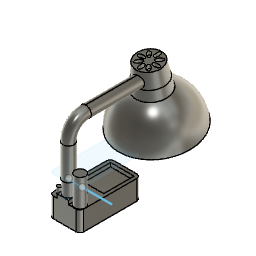
Project D1 (Autodesk Fusion 360 design; units mm, degrees)
Autodesk Fusion 360 part; units mm, degrees
sketch "Sketch1" plane through (0, 0, 0) normal (0, 1, 0) x (1, 0, 0)
sketch "Sketch2" plane through (0, 0, 0) normal (0, 0, 1) x (1, 0, 0)
  line L0 (0, 160) -> (80, 160)
  line L1 (80, 160) -> (80, 0)
  line L2 (80, 0) -> (0, 0)
  line L3 (0, 0) -> (0, 160)
  dimension "d1" = 80
  dimension "d2" = 160
  constraint horizontal L0
  constraint vertical L1
  constraint horizontal L2
  constraint vertical L3
  measures "d1" distance of L0.start L0.end
  measures "d2" distance of L0.start L2.end
extrude "Extrude1" add sketch "Sketch2" against normal blind 27 makes body 1
fillet "Fillet1" radius 10 3 edges at (80, 160, -13.5) (80, 0, -13.5) (0, 160, -13.5) on bodies 1
fillet "Fillet2" radius 10 1 edges at (0, 0, -13.5) on bodies 1
sketch "Sketch3" plane through (0, 0, 0) normal (0, 0, 1) x (-1, 0, 0)
  arc A0 (0, -10) -> (-10, 0) centre (-10, -10) ccw
  line L0 (-10, 0) -> (-70, 0)
  arc A1 (-70, 0) -> (-80, -10) centre (-70, -10) ccw
  line L1 (-80, -10) -> (-80, -150)
  arc A2 (-80, -150) -> (-70, -160) centre (-70, -150) ccw
  line L2 (-70, -160) -> (-10, -160)
  arc A3 (-10, -160) -> (0, -150) centre (-10, -150) ccw
  line L3 (0, -150) -> (0, -10)
sketch "Sketch4" plane through (0, 0, 0) normal (0, 0, 1) x (-1, 0, 0)
  line L0 (-71.3132, -71.4345) -> (-9.3132, -71.4345)
  line L1 (-9.3132, -71.4345) -> (-9.3132, -151.4345)
  line L2 (-9.3132, -151.4345) -> (-71.3132, -151.4345)
  line L3 (-71.3132, -151.4345) -> (-71.3132, -71.4345)
  dimension "d9" = 62
  dimension "d10" = 80
  constraint horizontal L0
  constraint vertical L1
  constraint horizontal L2
  constraint vertical L3
  measures "d9" distance of L0.start L0.end
  measures "d10" distance of L0.start L2.end
extrude "Extrude2" cut sketch "Sketch4" against normal blind 10 bodies 1
sketch "Sketch5" plane through (0, 0, 0) normal (0, 0, 1) x (1, 0, 0)
  circle A0 centre (65.5404, 14.9529) radius 14
  dimension "d13" = 28
  measures "d13" diameter of A0
extrude "Extrude3" add sketch "Sketch5" along normal blind 40 bodies 1
sketch "Sketch6" plane through (0, 0, 0) normal (0, 0, 1) x (1, 0, 0)
  line L0 (50, 0) -> (20, 0)
  line L1 (20, 0) -> (20, 50)
  line L2 (20, 50) -> (50, 50)
  line L3 (50, 50) -> (50, 0)
  dimension "d16" = 30
  constraint horizontal L0
  constraint vertical L1
  constraint horizontal L2
  constraint vertical L3
  measures "d16" distance of L0.start L0.end
extrude "Extrude4" add sketch "Sketch6" along normal blind 10 bodies 1
sketch "Sketch7" plane through (0, 0, 10) normal (0, 0, 1) x (-1, 0, 0)
  line L0 (-50, -50) -> (-20, -50)
  line L1 (-20, -50) -> (-20, 0)
  line L2 (-20, 0) -> (-50, 0)
  line L3 (-50, 0) -> (-50, -50)
  circle A0 centre (-35.247, -15.3012) radius 14
  dimension "d19" = 28
  measures "d19" diameter of A0
extrude "Extrude5" add sketch "Sketch7" along normal blind 15 contours A0 bodies 1
sketch "Sketch8" plane through (0, 0, 0) normal (0, 0, 1) x (1, 0, 0)
  circle A0 centre (10, 15) radius 5
  dimension "d22" = 10
  measures "d22" diameter of A0
extrude "Extrude6" add sketch "Sketch8" along normal blind 15 bodies 1
sketch "Sketch9" plane through (0, 0, 0) normal (0, 0, 1) x (1, 0, 0)
  line L0 (9.8673, 32.5058) -> (9.8673, 32.5058)
  line L1 (7.8673, 34.5058) -> (7.8673, 44.5058)
  line L2 (9.8673, 46.5058) -> (9.8673, 46.5058)
  line L3 (11.8673, 44.5058) -> (11.8673, 34.5058)
  arc A0 (9.8673, 32.5058) -> (11.8673, 34.5058) centre (9.8673, 34.5058) ccw
  arc A1 (7.8673, 34.5058) -> (9.8673, 32.5058) centre (9.8673, 34.5058) ccw
  arc A2 (11.8673, 44.5058) -> (9.8673, 46.5058) centre (9.8673, 44.5058) ccw
  arc A3 (9.8673, 46.5058) -> (7.8673, 44.5058) centre (9.8673, 44.5058) ccw
  point P0 (11.8673, 32.5058)
  point P1 (7.8673, 32.5058)
  point P2 (11.8673, 46.5058)
  dimension "d25" = 4
  dimension "d26" = 14
  dimension "d27" = 2
  dimension "d28" = 2
  dimension "d29" = 2
  constraint vertical L1
  constraint vertical L3
  constraint coincident P0 L3
  constraint tangent L3 A0
  constraint coincident P1 L0
  constraint coincident P1 L1
  constraint tangent L1 A1
  constraint coincident P2 L3
  constraint tangent L3 A2
  constraint tangent L1 A3
  constraint equal A2 A3
  measures "d25" distance of P0 P1
  measures "d26" distance of P0 P2
  measures "d27" radius of A0
  measures "d28" radius of A1
  measures "d29" radius of A2
extrude "Extrude7" cut sketch "Sketch9" against normal blind 7 bodies 1
sketch "Sketch10" plane through (0, 0, 10) normal (0, 0, 1) x (-1, 0, 0)
  circle A0 centre (-35.247, -15.3012) radius 14
  line L0 (-50, -50) -> (-20, -50)
  line L1 (-20, -50) -> (-20, 0)
  line L2 (-20, 0) -> (-50, 0)
  line L3 (-50, 0) -> (-50, -50)
  line L4 (-31, -45) -> (-39, -45)
  line L5 (-39, -45) -> (-39, -35)
  line L6 (-39, -35) -> (-31, -35)
  line L7 (-31, -35) -> (-31, -45)
  dimension "d32" = 8
  dimension "d33" = 10
  constraint horizontal L4
  constraint vertical L5
  constraint horizontal L6
  constraint vertical L7
  measures "d32" distance of L4.start L4.end
  measures "d33" distance of L4.start L6.end
extrude "Extrude8" cut sketch "Sketch10" against normal blind 7 contours L4 L5 L6 L7 bodies 1
sketch "Sketch11" plane through (0, 0, 0) normal (1, 0, 0) x (0, 1, 0)
  line L0 (16.2634, 104.9165) -> (1.2634, 104.9165)
  line L1 (1.2634, 104.9165) -> (1.2634, 39.9165)
  line L2 (1.2634, 39.9165) -> (16.2634, 39.9165)
  line L3 (16.2634, 39.9165) -> (16.2634, 104.9165)
  line L4 (16.2634, 110.373) -> (16.2634, 35)
  dimension "d36" = 15
  dimension "d37" = 65
  constraint horizontal L0
  constraint vertical L1
  constraint horizontal L2
  constraint vertical L3
  constraint perpendicular L2 L4
  measures "d36" distance of L0.start L0.end
  measures "d37" distance of L0.start L2.end
revolve "Revolve1" add sketch "Sketch11" angle 360 about axis through (0, 16.2634, 110.373) along (0, 0, -1) separate body makes body 2
move_face "MoveFace1" to x (1, 0, 0) y (0, 1, 0) z (0, 0, 1) at (40, 0, 10) 1 faces at (0.7477, 1.282, 83.2498) on bodies 2
move_body "Move1" bodies 2 to x (1, 0, 0) y (0, 1, 0) z (0, 0, 1) at (-5, 0, -20)
sketch "Sketch12" plane through (0, 0, 0) normal (1, 0, 0) x (0, 1, 0)
sketch "Sketch13" plane through (0, 0, 0) normal (1, 0, 0) x (0, 1, 0)
sketch "Sketch14" plane through (0, 0, 0) normal (1, 0, 0) x (0, 1, 0)
  arc A0 (60, 122.9657) -> (17.0403, 79.284) centre (60, 80) ccw
pipe "Pipe1" add diameter 30 path "Sketch14" along A0 separate body makes body 3
move_face "MoveFace2" to x (1, 0, 0) y (0, 1, 0) z (0, 0, 1) at (0, -1, 0) 1 faces at (35.7477, 1.282, 63.2498) on bodies 2
move_face "MoveFace3" to x (1, 0, 0) y (0, 1, 0) z (0, 0, 1) at (0, -2, 2) 1 faces at (4.0626, 6.6698, 101.2421) on bodies 3
move_face "MoveFace4" to x (1, 0, 0) y (0, 1, 0) z (0, 0, 1) at (35, 0, 0) 1 faces at (-1.7653, 54.7653, 139.771) on bodies 3
extrude "Extrude9" add 1 faces at (30.0178, 60, 124.8543) along direction (0, 1, 0) blind 90 on bodies 3 bodies 3
extrude "Extrude10" add 1 faces at (26.6667, 56.6667, -27) along direction (0, 0, -1) blind 25 on bodies 1 bodies 1
sketch "Sketch15" plane through (0, 0, 0) normal (1, 0, 0) x (0, 1, 0)
sketch "Sketch16" plane through (0, 0, 0) normal (1, 0, 0) x (0, 1, 0)
  line L0 (282.5766, 151.0827) -> (279.0659, 177.8527)
  line L1 (282.5766, 151.0827) -> (308.0478, 151.0827) construction
  line L2 (279.0659, 177.8527) -> (273.8459, 217.5027)
  line L3 (279.0659, 177.8527) -> (317.4124, 177.8527) construction
  arc A0 (340, 60) -> (240, 160) centre (240, 60) ccw
  line L4 (240, 160) -> (240, 60)
  line L5 (240, 60) -> (340, 60)
  line L6 (282.5766, 151.0827) -> (240, 151.0827)
  line L7 (240, 180) -> (278.7832, 180)
  line L8 (273.8459, 217.5027) -> (240, 217.5027)
  line L9 (240, 217.5027) -> (240, 180)
  line L10 (240, 180) -> (240, 151.0827)
  line L11 (240, 240) -> (240, 50)
  dimension "d72" = 26.77
  constraint horizontal L1
  constraint horizontal L3
  constraint coincident A0.centre L4.end
  constraint perpendicular L4 L5
  constraint coincident L4 L6.end
  constraint perpendicular L4 L6
  constraint coincident L2 L7.end
  constraint parallel L6 L7
  constraint perpendicular L4 L8
  constraint perpendicular L7 L9
  constraint perpendicular L6 L10
  constraint perpendicular L5 L11
  measures "d72" vertical distance of L0.start L0.end
revolve "Revolve2" add sketch "Sketch16" angle 360 about axis through (0, 240, 240) along (0, 0, -1) separate body makes body 4
move_body "Move2" bodies 4 to x (1, 0, 0) y (0, 0.976296, 0.21644) z (0, -0.21644, 0.976296) at (0, 47.0867, -113.4516)
move_body "Move3" bodies 4 to x (1, 0, 0) y (0, 0.996195, -0.087156) z (0, 0.087156, 0.996195) at (0, 2.7825, 14.5845)
move_body "Move4" bodies 4 to x (1, 0, 0) y (0, 1, 0) z (0, 0, 1) at (0, -70, 10)
move_body "Move5" bodies 4 to x (1, 0, 0) y (0, 1, 0) z (0, 0, 1) at (32, 0, 0)
move_body "Move6" bodies 1 to x (1, 0, 0) y (0, 1, 0) z (0, 0, 1) at (0, 0, -50)
move_body "Move7" bodies 2 to x (1, 0, 0) y (0, 1, 0) z (0, 0, 1) at (0, 0, -25)
extrude "Extrude11" add 1 faces at (38.3611, 9.7448, 59.9165) along direction (0, 0, 1) blind 20 on bodies 2 bodies 2 4 3
move_body "Move8" bodies 4 to x (1, 0, 0) y (0, 1, 0) z (0, 0, 1) at (0, 50, 0)
extrude "Extrude12" add 1 faces at (67.8737, 10.9115, -10) along direction (0, 0, 1) blind 7 on bodies 1 bodies 1
extrude "Extrude13" add 1 faces at (30.0178, 150, 124.8543) along direction (0, 1, 0) blind 50 on bodies 2 bodies 2 4
sketch "Sketch17" plane through (0, -16.077, 122.1167) normal (0, -0.130526, 0.991445) x (1, 0, 0)
  circle A0 centre (32, 247.5539) radius 33.8459
  ellipse E0 centre (12.5438, 247.5239) end of major axis (22.1005, 247.5239) minor radius 5
  line L0 (2.987, 247.5239) -> (22.1005, 247.5239)
  line L1 (12.5438, 242.5239) -> (12.5438, 252.5239)
  dimension "d83" = 10
  constraint coincident E0 L0.start
  constraint coincident E0 L0.end
  constraint coincident E0 L1.start
  constraint coincident E0 L1.end
sketch "Sketch18" plane through (32, 229.359, 154.4289) normal (0, -0.130526, 0.991445) x (1, 0, 0)
extrude "Extrude14" add 1 faces at (39.8615, 9.6484, -25) along direction (0, 0, 1) blind 22 on bodies 1 bodies 1 2
extrude "Extrude15" add 1 faces at (67.8737, 10.9115, -3) along direction (0, 0, 1) blind 25 on bodies 1 bodies 1
sketch "Sketch19" plane through (0, 0, -40) normal (0, 0, 1) x (-1, 0, 0)
  line L0 (-39, -45) -> (-39, -35)
  line L1 (-39, -35) -> (-31, -35)
  line L2 (-31, -35) -> (-31, -45)
  line L3 (-31, -45) -> (-39, -45)
  circle A0 centre (-35.247, -15.3012) radius 14
  line L4 (-50, -50) -> (-20, -50)
  line L5 (-20, -50) -> (-20, 0)
  line L6 (-20, 0) -> (-50, 0)
  line L7 (-50, 0) -> (-50, -50)
  line L8 (0, -50) -> (0, -47.6437)
  line L9 (0, -47.6437) -> (-114.7068, -47.6437)
  line L10 (-114.7068, -47.6437) -> (-38.5734, -47.6437)
  constraint vertical L8
  constraint perpendicular L8 L9
  constraint parallel L9 L10
sketch "Sketch20" plane through (0, 0, 0) normal (0, 0, 1) x (1, 0, 0)
sketch "Sketch21" plane through (0, 0, 0) normal (1, 0, 0) x (0, 1, 0)
  line L0 (40, -30) -> (37.0787, -33.5355)
  arc A0 (40, -30) -> (45, -32.831) centre (45, -27) ccw
  line L1 (45, -32.831) -> (45, -36)
  line L2 (45, -36) -> (37, -36)
  line L3 (37, -36) -> (37.0787, -33.5355)
  constraint vertical L1
  constraint perpendicular L1 L2
extrude "Extrude16" add sketch "Sketch21" along normal blind 10 separate body makes body 5
move_body "Move9" bodies 5 to x (1, 0, 0) y (0, 1, 0) z (0, 0, 1) at (30, 0, -5.5)
sketch "Sketch22" plane through (32, 229.359, 154.4289) normal (0, -0.130526, 0.991445) x (1, 0, 0)
extrude "Extrude17" add sketch "Sketch17" along normal blind 1 contours E0 L0 L1 | E0 L0 L1 | E0 L0 L1 | E0 L0 L1 bodies 1
sketch "Sketch23" plane through (0, -16.077, 122.1167) normal (0, -0.130526, 0.991445) x (1, 0, 0)
  ellipse E0 centre (12.5438, 247.5239) end of major axis (22.1005, 247.5239) minor radius 5
  circle A0 centre (32, 247.5539) radius 33.8459
  ellipse E1 centre (52.1147, 247.0081) end of major axis (42.1147, 247.0081) minor radius 5
  line L0 (62.1147, 247.0081) -> (42.1147, 247.0081)
  line L1 (52.1147, 252.0081) -> (52.1147, 242.0081)
  ellipse E2 centre (18.9077, 260.8879) end of major axis (25.6653, 254.1303) minor radius 5
  ellipse E3 centre (32.3427, 270.0803) end of major axis (32.3427, 260.5236) minor radius 5
  ellipse E4 centre (46.1147, 262.0081) end of major axis (39.0436, 254.937) minor radius 5
  line L2 (53.1858, 269.0792) -> (39.0436, 254.937)
  line L3 (42.5792, 265.5436) -> (49.6502, 258.4726)
  ellipse E5 centre (32.3427, 227.0803) end of major axis (32.3427, 217.5236) minor radius 5
  ellipse E6 centre (18.1147, 234.0081) end of major axis (11.0436, 226.937) minor radius 5
  line L4 (25.1858, 241.0792) -> (11.0436, 226.937)
  line L5 (14.5792, 237.5436) -> (21.6502, 230.4726)
  ellipse E7 centre (45.9077, 232.8879) end of major axis (52.6653, 226.1303) minor radius 5
  dimension "d95" = 20
  dimension "d96" = 20
  dimension "d97" = 20
  constraint horizontal L0
  constraint coincident E1 L0.start
  constraint coincident E1 L0.end
  constraint coincident E1 L1.start
  constraint coincident E1 L1.end
  constraint coincident E4 L2.start
  constraint coincident E4 L2.end
  constraint coincident E4 L3.start
  constraint coincident E4 L3.end
  constraint coincident E6 L4.start
  constraint coincident E6 L4.end
  constraint coincident E6 L5.start
  constraint coincident E6 L5.end
  measures "d95" distance of E1
  measures "d96" distance of E4
  measures "d97" distance of E6
extrude "Extrude18" cut sketch "Sketch23" against normal blind 10 contours E1 L0 L1 | E1 L0 L1 | E1 L0 L1 | E1 L0 L1 | E2 | E3 | E4 L2 L3 | E4 L2 L3 | E4 L2 L3 | E4 L2 L3 | E5 | E6 L4 L5 | E6 L4 L5 | E6 L4 L5 | E6 L4 L5 | E7 bodies 1
extrude "Extrude19" cut 1 faces at (11.4176, 230.8024, 155.6276) along direction (0, 0.130526, -0.991445) blind 10 on bodies 1 bodies 1
